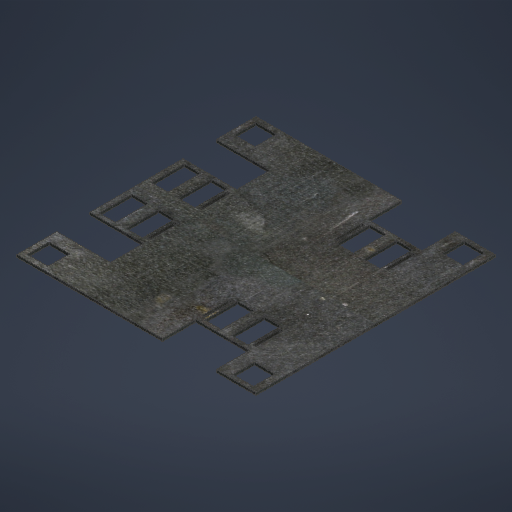
# Autodesk Inventor part: base2
Saved by Autodesk Inventor 2026.2 (Build 302298010, 298A)
## iProperties
Created: 2026-09-07
Part Number: base2
Material: Steel
Document SubType Name: Modeling
Designer: karol
Density: 7.85 g/cm^3
Appearance: Plate
Author: karol
Autodesk Inventor part; units mm, degrees
ref_plane "YZ Plane" through (0, 0, 0) normal (1, 0, 0) x (0, 1, 0)
ref_plane "XZ Plane" through (0, 0, 0) normal (0, 1, 0) x (-1, 0, 0)
ref_plane "XY Plane" through (0, 0, 0) normal (0, 0, 1) x (1, 0, 0)
sketch "Sketch1" plane through (0, 0, 0) normal (0, 1, 0) x (-1, 0, 0)
  line L0 (180, 90) -> (0, 90)
  line L1 (0, 90) -> (0, -90)
  line L2 (0, -90) -> (180, -90)
  line L3 (180, -90) -> (180, 90)
  line L4 (0, -0.2542) -> (0, 0)
  line L5 (0, 0) -> (0, 6.4289)
  line L6 (0, 0) -> (28.373, 0)
  line L7 (177, 0) -> (135, 0)
  line L8 (135, 0) -> (135, -7.5)
  line L9 (135, -7.5) -> (177, -7.5)
  line L10 (177, -7.5) -> (177, 0)
  line L11 (177, 0) -> (180, 0)
  line L12 (180, 0) -> (180, -35)
  line L13 (180, -35) -> (177, -35)
  line L14 (177, -35) -> (177, 0)
  line L15 (180, -35) -> (136.6, -35)
  line L16 (136.6, -35) -> (136.6, -32)
  line L17 (136.6, -32) -> (180, -32)
  line L18 (180, -32) -> (180, -35)
  line L19 (177, -7.5) -> (176, -7.5)
  line L20 (176, -7.5) -> (176, -32)
  line L21 (176, -32) -> (177, -32)
  line L22 (177, -32) -> (177, -7.5)
  line L23 (176, -7.5) -> (163.8, -7.5)
  line L24 (163.8, -7.5) -> (163.8, -32)
  line L25 (163.8, -32) -> (176, -32)
  line L26 (176, -32) -> (176, -7.5)
  line L27 (163.8, -7.5) -> (159.8, -7.5)
  line L28 (159.8, -7.5) -> (159.8, -32)
  line L29 (159.8, -32) -> (163.8, -32)
  line L30 (163.8, -32) -> (163.8, -7.5)
  line L31 (159.8, -7.5) -> (155.8, -7.5)
  line L32 (155.8, -7.5) -> (155.8, -32)
  line L33 (155.8, -32) -> (159.8, -32)
  line L34 (159.8, -32) -> (159.8, -7.5)
  line L35 (155.8, -7.5) -> (143.6, -7.5)
  line L36 (143.6, -7.5) -> (143.6, -32)
  line L37 (143.6, -32) -> (155.8, -32)
  line L38 (155.8, -32) -> (155.8, -7.5)
  line L39 (143.6, -7.5) -> (139.6, -7.5)
  line L40 (139.6, -7.5) -> (139.6, -32)
  line L41 (139.6, -32) -> (143.6, -32)
  line L42 (143.6, -32) -> (143.6, -7.5)
  line L43 (136.6, -35) -> (139.6, -35)
  line L44 (139.6, -35) -> (139.6, -32)
  line L45 (139.6, -32) -> (136.6, -32)
  line L46 (136.6, -32) -> (136.6, -35)
  line L47 (139.6, -35) -> (136.6, -35)
  line L48 (136.6, -35) -> (136.6, -60)
  line L49 (136.6, -60) -> (139.6, -60)
  line L50 (139.6, -60) -> (139.6, -35)
  line L51 (136.6, -60) -> (180, -60)
  line L52 (180, -60) -> (180, -63)
  line L53 (180, -63) -> (136.6, -63)
  line L54 (136.6, -63) -> (136.6, -60)
  line L55 (180, -63) -> (176, -63)
  line L56 (176, -63) -> (176, -90)
  line L57 (176, -90) -> (180, -90)
  line L58 (180, -90) -> (180, -63)
  line L59 (163.8, -7.5) -> (169.9, -7.5)
  line L60 (169.9, -7.5) -> (169.9, -32)
  line L61 (169.9, -32) -> (163.8, -32)
  line L62 (163.8, -32) -> (163.8, -7.5)
  line L63 (143.6, -7.5) -> (149.7, -7.5)
  line L64 (149.7, -7.5) -> (149.7, -32)
  line L65 (149.7, -32) -> (143.6, -32)
  line L66 (143.6, -32) -> (143.6, -7.5)
  line L67 (176, -90) -> (73.4, -90)
  line L68 (73.4, -90) -> (73.4, -86)
  line L69 (73.4, -86) -> (176, -86)
  line L70 (176, -86) -> (176, -90)
  line L71 (176, -86) -> (160.6, -86)
  line L72 (160.6, -86) -> (160.6, -69.8)
  line L73 (160.6, -69.8) -> (176, -69.8)
  line L74 (176, -69.8) -> (176, -86)
  line L75 (70.4, -90) -> (30, -90)
  line L76 (27, -90) -> (0, -90)
  line L77 (0, -90) -> (0, -87)
  line L78 (70.4, -90) -> (73.4, -90)
  line L79 (0, -90) -> (30, -90)
  line L80 (30, -90) -> (30, -87)
  line L81 (30, -87) -> (0, -87)
  line L82 (0, -87) -> (0, -90)
  line L83 (30, -87) -> (27, -87)
  line L84 (27, -87) -> (27, -65)
  line L85 (27, -65) -> (30, -65)
  line L86 (30, -65) -> (30, -87)
  line L87 (27, -65) -> (73.4, -65)
  line L88 (73.4, -65) -> (73.4, -62)
  line L89 (73.4, -62) -> (27, -62)
  line L90 (27, -62) -> (27, -65)
  line L91 (73.4, -62) -> (70.4, -62)
  line L92 (70.4, -62) -> (70.4, -90)
  line L93 (70.4, -90) -> (73.4, -90)
  line L94 (73.4, -90) -> (73.4, -62)
  line L95 (30, -90) -> (24, -90)
  line L96 (24, -90) -> (24, -84)
  line L97 (24, -84) -> (30, -84)
  line L98 (30, -84) -> (30, -90)
  line L99 (73.4, -62) -> (66.4, -62)
  line L100 (66.4, -62) -> (66.4, -37.5)
  line L101 (66.4, -37.5) -> (73.4, -37.5)
  line L102 (73.4, -37.5) -> (73.4, -62)
  line L103 (66.4, -37.5) -> (54.2, -37.5)
  line L104 (54.2, -37.5) -> (54.2, -62)
  line L105 (54.2, -62) -> (66.4, -62)
  line L106 (66.4, -62) -> (66.4, -37.5)
  line L107 (54.2, -37.5) -> (50.2, -37.5)
  line L108 (50.2, -37.5) -> (50.2, -62)
  line L109 (50.2, -62) -> (54.2, -62)
  line L110 (54.2, -62) -> (54.2, -37.5)
  line L111 (50.2, -37.5) -> (46.2, -37.5)
  line L112 (46.2, -37.5) -> (46.2, -62)
  line L113 (46.2, -62) -> (50.2, -62)
  line L114 (50.2, -62) -> (50.2, -37.5)
  line L115 (46.2, -37.5) -> (34, -37.5)
  line L116 (34, -37.5) -> (34, -62)
  line L117 (34, -62) -> (46.2, -62)
  line L118 (46.2, -62) -> (46.2, -37.5)
  line L119 (34, -37.5) -> (27, -37.5)
  line L120 (27, -37.5) -> (27, -62)
  line L121 (27, -62) -> (34, -62)
  line L122 (34, -62) -> (34, -37.5)
  line L123 (5, -87) -> (20.4, -87)
  line L124 (20.4, -87) -> (20.4, -70.8)
  line L125 (20.4, -70.8) -> (5, -70.8)
  line L126 (5, -70.8) -> (5, -87)
  line L127 (0, 90) -> (180, 90)
  line L128 (135, 7.5) -> (177, 7.5)
  line L129 (180, 35) -> (177, 35)
  line L130 (180, 35) -> (136.6, 35)
  line L131 (136.6, 35) -> (136.6, 32)
  line L132 (136.6, 32) -> (180, 32)
  line L133 (180, 32) -> (180, 35)
  line L134 (177, 7.5) -> (176, 7.5)
  line L135 (176, 7.5) -> (176, 32)
  line L136 (176, 32) -> (177, 32)
  line L137 (177, 32) -> (177, 7.5)
  line L138 (176, 7.5) -> (163.8, 7.5)
  line L139 (163.8, 7.5) -> (163.8, 32)
  line L140 (163.8, 32) -> (176, 32)
  line L141 (176, 32) -> (176, 7.5)
  line L142 (163.8, 7.5) -> (159.8, 7.5)
  line L143 (159.8, 7.5) -> (159.8, 32)
  line L144 (159.8, 32) -> (163.8, 32)
  line L145 (163.8, 32) -> (163.8, 7.5)
  line L146 (159.8, 7.5) -> (155.8, 7.5)
  line L147 (155.8, 7.5) -> (155.8, 32)
  line L148 (155.8, 32) -> (159.8, 32)
  line L149 (159.8, 32) -> (159.8, 7.5)
  line L150 (155.8, 7.5) -> (143.6, 7.5)
  line L151 (143.6, 7.5) -> (143.6, 32)
  line L152 (143.6, 32) -> (155.8, 32)
  line L153 (155.8, 32) -> (155.8, 7.5)
  line L154 (143.6, 7.5) -> (139.6, 7.5)
  line L155 (139.6, 7.5) -> (139.6, 32)
  line L156 (139.6, 32) -> (143.6, 32)
  line L157 (143.6, 32) -> (143.6, 7.5)
  line L158 (136.6, 35) -> (139.6, 35)
  line L159 (139.6, 35) -> (139.6, 32)
  line L160 (139.6, 32) -> (136.6, 32)
  line L161 (136.6, 32) -> (136.6, 35)
  line L162 (139.6, 35) -> (136.6, 35)
  line L163 (136.6, 35) -> (136.6, 60)
  line L164 (136.6, 60) -> (139.6, 60)
  line L165 (139.6, 60) -> (139.6, 35)
  line L166 (136.6, 60) -> (180, 60)
  line L167 (180, 60) -> (180, 63)
  line L168 (180, 63) -> (136.6, 63)
  line L169 (136.6, 63) -> (136.6, 60)
  line L170 (180, 63) -> (176, 63)
  line L171 (176, 63) -> (176, 90)
  line L172 (176, 90) -> (180, 90)
  line L173 (180, 90) -> (180, 63)
  line L174 (163.8, 7.5) -> (169.9, 7.5)
  line L175 (169.9, 7.5) -> (169.9, 32)
  line L176 (169.9, 32) -> (163.8, 32)
  line L177 (163.8, 32) -> (163.8, 7.5)
  line L178 (143.6, 7.5) -> (149.7, 7.5)
  line L179 (149.7, 7.5) -> (149.7, 32)
  line L180 (149.7, 32) -> (143.6, 32)
  line L181 (143.6, 32) -> (143.6, 7.5)
  line L182 (176, 90) -> (73.4, 90)
  line L183 (73.4, 90) -> (73.4, 86)
  line L184 (73.4, 86) -> (176, 86)
  line L185 (176, 86) -> (176, 90)
  line L186 (176, 86) -> (160.6, 86)
  line L187 (160.6, 86) -> (160.6, 69.8)
  line L188 (160.6, 69.8) -> (176, 69.8)
  line L189 (176, 69.8) -> (176, 86)
  line L190 (70.4, 90) -> (30, 90)
  line L191 (27, 90) -> (0, 90)
  line L192 (0, 90) -> (0, 87)
  line L193 (70.4, 90) -> (73.4, 90)
  line L194 (0, 90) -> (30, 90)
  line L195 (30, 90) -> (30, 87)
  line L196 (30, 87) -> (0, 87)
  line L197 (0, 87) -> (0, 90)
  line L198 (30, 87) -> (27, 87)
  line L199 (27, 87) -> (27, 65)
  line L200 (27, 65) -> (30, 65)
  line L201 (30, 65) -> (30, 87)
  line L202 (27, 65) -> (73.4, 65)
  line L203 (73.4, 65) -> (73.4, 62)
  line L204 (73.4, 62) -> (27, 62)
  line L205 (27, 62) -> (27, 65)
  line L206 (73.4, 62) -> (70.4, 62)
  line L207 (70.4, 62) -> (70.4, 90)
  line L208 (70.4, 90) -> (73.4, 90)
  line L209 (73.4, 90) -> (73.4, 62)
  line L210 (30, 90) -> (24, 90)
  line L211 (24, 90) -> (24, 84)
  line L212 (24, 84) -> (30, 84)
  line L213 (30, 84) -> (30, 90)
  line L214 (73.4, 62) -> (66.4, 62)
  line L215 (66.4, 62) -> (66.4, 37.5)
  line L216 (66.4, 37.5) -> (73.4, 37.5)
  line L217 (73.4, 37.5) -> (73.4, 62)
  line L218 (66.4, 37.5) -> (54.2, 37.5)
  line L219 (54.2, 37.5) -> (54.2, 62)
  line L220 (54.2, 62) -> (66.4, 62)
  line L221 (66.4, 62) -> (66.4, 37.5)
  line L222 (54.2, 37.5) -> (50.2, 37.5)
  line L223 (50.2, 37.5) -> (50.2, 62)
  line L224 (50.2, 62) -> (54.2, 62)
  line L225 (54.2, 62) -> (54.2, 37.5)
  line L226 (50.2, 37.5) -> (46.2, 37.5)
  line L227 (46.2, 37.5) -> (46.2, 62)
  line L228 (46.2, 62) -> (50.2, 62)
  line L229 (50.2, 62) -> (50.2, 37.5)
  line L230 (46.2, 37.5) -> (34, 37.5)
  line L231 (34, 37.5) -> (34, 62)
  line L232 (34, 62) -> (46.2, 62)
  line L233 (46.2, 62) -> (46.2, 37.5)
  line L234 (34, 37.5) -> (27, 37.5)
  line L235 (27, 37.5) -> (27, 62)
  line L236 (27, 62) -> (34, 62)
  line L237 (34, 62) -> (34, 37.5)
  line L238 (5, 87) -> (20.4, 87)
  line L239 (20.4, 87) -> (20.4, 70.8)
  line L240 (20.4, 70.8) -> (5, 70.8)
  line L241 (5, 70.8) -> (5, 87)
  line L242 (177, 7.5) -> (135, 7.5)
  line L243 (135, 7.5) -> (135, 0)
  line L244 (135, 0) -> (177, 0)
  line L245 (177, 0) -> (177, 7.5)
  point P0 (177, -3.75)
  point P1 (177, 3.75)
  point P2 (70.4, 65)
  point P3 (70.4, -65)
  dimension "d2" = 180
  dimension "d3" = 180
  dimension "d4" = 90
  dimension "d5" = 42
  dimension "d6" = 7.5
  dimension "d7" = 3
  dimension "d8" = 35
  dimension "d9" = 3
  dimension "d10" = 1
  dimension "d11" = 12.2
  dimension "d12" = 4
  dimension "d13" = 4
  dimension "d14" = 12.2
  dimension "d15" = 4
  dimension "d16" = 25
  dimension "d17" = 3
  dimension "d18" = 3
  dimension "d19" = 4
  dimension "d20" = 102.6
  dimension "d22" = 15.4
  dimension "d23" = 16.2
  dimension "d42" = 30
  dimension "d43" = 3
  dimension "d44" = 22
  dimension "d46" = 3
  dimension "d47" = 3
  dimension "d48" = 6
  dimension "d49" = 6
  dimension "d50" = 7
  dimension "d51" = 24.5
  dimension "d52" = 12.2
  dimension "d53" = 4
  dimension "d54" = 4
  dimension "d55" = 12.2
  dimension "d56" = 7
  dimension "d57" = 3
  dimension "d58" = 4
  dimension "d59" = 15.4
  dimension "d60" = 16.2
  dimension "d61" = 5
  constraints: 492 end point, 93 symmetric about line, 62 parallel, 35 point on line, 34 horizontal, 32 perpendicular, 5 midpoint, 1 collinear, 1 vertical
  measures "d2" distance of L2.end L1.end
  measures "d3" distance of L1.end L0.end
  measures "d4" distance between parallel lines of L0 L6
  measures "d5" distance of L9.end L8.end
  measures "d6" distance of L8.end L7.end
  measures "d7" distance from line of L3 point (177, -3.75)
  measures "d8" distance of L11.end L12.end
  measures "d9" distance of L15.end L16.end
  measures "d10" distance of L21.end L20.end
  measures "d11" distance of L25.end L24.end
  measures "d12" distance of L29.end L28.end
  measures "d13" distance of L33.end L32.end
  measures "d14" distance of L37.end L36.end
  measures "d15" distance of L41.end L40.end
  measures "d16" distance of L48.end L47.end
  measures "d17" distance of L51.end L52.end
  measures "d18" distance between parallel lines of L48 L50
  measures "d19" distance between parallel lines of L3 L56
  measures "d20" distance of L68.end L69.end
  measures "d22" distance of L72.end L73.end
  measures "d23" distance of L71.end L72.end
  measures "d42" distance of L81.end L80.end
  measures "d43" distance of L80.end L79.end
  measures "d44" distance of L83.end L84.end
  measures "d46" distance of L88.end L87.end
  measures "d47" distance of L93.end L92.end
  measures "d48" distance of L96.end L97.end
  measures "d49" distance of L95.end L96.end
  measures "d50" distance of L100.end L101.end
  measures "d51" distance of L99.end L100.end
  measures "d52" distance of L105.end L104.end
  measures "d53" distance of L109.end L108.end
  measures "d54" distance of L113.end L112.end
  measures "d55" distance of L117.end L116.end
  measures "d56" distance between parallel lines of L116 L120
  measures "d57" distance between parallel lines of L98 L84
  measures "d58" distance between parallel lines of L67 L69
  measures "d59" distance of L125.end L124.end
  measures "d60" distance of L124.end L123.end
  measures "d61" distance between parallel lines of L126 L1
extrude "Extrusion1" add sketch "Sketch1" along normal blind 2 contours L3 L168 L171 L0 | L171 L184 L183 L0 | L3 L166 L164 L169 L168 | L183 L209 L202 L207 L0 | L168 L169 L163 L131 L132 L155 L128 L243 L8 L9 L40 L17 L16 L48 L54 L53 L56 L73 L72 L69 L94 L88 L102 L101 L103 L107 L111 L115 L119 L120 L90 L84 L97 L96 L81 L124 L125 L126 L1 L196 L241 L240 L239 L211 L212 L199 L205 L235 L234 L230 L226 L222 L218 L216 L217 L203 L209 L184 L187 L188 L171 | L3 L132 L159 L130 L129 | L165 L130 L163 L164 | L195 L196 L211 L0 | L207 L204 L205 L200 L202 | L202 L203 L204 L207 | L3 L11 L245 L137 L132 | L159 L132 L131 L130 | L201 L212 L199 L196 | L200 L199 L212 L201 | L204 L217 L216 L215 | L3 L17 L14 L10 L11 | L137 L128 L135 L132 | L132 L151 L128 L155 | L211 L196 L1 L0 | L199 L212 L211 L196 | L3 L13 L14 L17 | L10 L9 L8 L7 | L7 L243 L128 L245 | L204 L231 L234 L235 | L219 L222 L223 L204 | L17 L20 L9 L14 | L14 L15 L44 L17 | L223 L226 L227 L204 | L3 L53 L54 L49 L51 | L139 L128 L143 L132 | L132 L143 L128 L147 | L3 L2 L56 L53 | L49 L48 L15 L50 | L15 L16 L17 L44 | L9 L36 L17 L40 | L17 L28 L9 L24 | L2 L68 L69 L56 | L17 L32 L9 L28 | L81 L96 L2 L1 | L2 L92 L87 L94 L68 | L96 L81 L80 L2 | L92 L89 L88 L87 | L87 L85 L90 L89 L92 | L96 L97 L84 L81 | L81 L84 L97 L86 | L86 L97 L84 L85 | L89 L100 L101 L102 | L120 L119 L116 L89 | L89 L108 L107 L104 | L89 L112 L111 L108
sketch "Sketch2" plane through (0, 0, 0) normal (0, -1, 0) x (1, 0, 0)
  line L0 (-143.6, -7.5) -> (-155.8, -7.5) projected
  line L1 (-143.6, -7.5) -> (-141.6, -7.5)
  line L2 (-141.6, -7.5) -> (-141.6, -32)
  line L3 (-141.6, -32) -> (-143.6, -32)
  line L4 (-143.6, -32) -> (-143.6, -7.5)
  line L5 (-143.6, 7.5) -> (-143.6, 32) projected
  line L6 (-143.6, 32) -> (-141.6, 32)
  line L7 (-141.6, 32) -> (-141.6, 7.5)
  line L8 (-141.6, 7.5) -> (-143.6, 7.5)
  line L9 (-143.6, 7.5) -> (-143.6, 32)
  line L10 (-141.6, 32) -> (-139.6, 32)
  line L11 (-139.6, 32) -> (-139.6, 7.5)
  line L12 (-139.6, 7.5) -> (-141.6, 7.5)
  line L13 (-141.6, 7.5) -> (-141.6, 32)
  line L14 (-141.6, -7.5) -> (-139.6, -7.5)
  line L15 (-139.6, -7.5) -> (-139.6, -32)
  line L16 (-139.6, -32) -> (-141.6, -32)
  line L17 (-141.6, -32) -> (-141.6, -7.5)
  line L18 (-66.4, 62) -> (-66.4, 37.5) projected
  line L19 (-66.4, 62) -> (-68.4, 62)
  line L20 (-68.4, 62) -> (-68.4, 37.5)
  line L21 (-68.4, 37.5) -> (-66.4, 37.5)
  line L22 (-66.4, 37.5) -> (-66.4, 62)
  line L23 (-34, 37.5) -> (-34, 62) projected
  line L24 (-34, 62) -> (-32, 62)
  line L25 (-32, 62) -> (-32, 37.5)
  line L26 (-32, 37.5) -> (-34, 37.5)
  line L27 (-34, 37.5) -> (-34, 62)
  line L28 (-32, 62) -> (-30, 62)
  line L29 (-30, 62) -> (-30, 37.5)
  line L30 (-30, 37.5) -> (-32, 37.5)
  line L31 (-32, 37.5) -> (-32, 62)
  line L32 (-68.4, 62) -> (-70.4, 62)
  line L33 (-70.4, 62) -> (-70.4, 37.5)
  line L34 (-70.4, 37.5) -> (-68.4, 37.5)
  line L35 (-68.4, 37.5) -> (-68.4, 62)
  line L36 (-34, -37.5) -> (-46.2, -37.5) projected
  line L37 (-34, -37.5) -> (-32, -37.5)
  line L38 (-32, -37.5) -> (-32, -62)
  line L39 (-32, -62) -> (-34, -62)
  line L40 (-34, -62) -> (-34, -37.5)
  line L41 (-32, -62) -> (-30, -62)
  line L42 (-30, -62) -> (-30, -37.5)
  line L43 (-30, -37.5) -> (-32, -37.5)
  line L44 (-32, -37.5) -> (-32, -62)
  line L45 (-54.2, -37.5) -> (-66.4, -37.5) projected
  line L46 (-66.4, -37.5) -> (-68.4, -37.5)
  line L47 (-68.4, -37.5) -> (-68.4, -62)
  line L48 (-68.4, -62) -> (-66.4, -62)
  line L49 (-66.4, -62) -> (-66.4, -37.5)
  line L50 (-68.4, -62) -> (-70.4, -62)
  line L51 (-70.4, -62) -> (-70.4, -37.5)
  line L52 (-70.4, -37.5) -> (-68.4, -37.5)
  line L53 (-68.4, -37.5) -> (-68.4, -62)
  line L54 (-70.4, -37.5) -> (-66.4, -37.5)
  line L55 (-66.4, -37.5) -> (-66.4, -39.5)
  line L56 (-66.4, -39.5) -> (-70.4, -39.5)
  line L57 (-70.4, -39.5) -> (-70.4, -37.5)
  line L58 (-66.4, -62) -> (-70.4, -62)
  line L59 (-70.4, -62) -> (-70.4, -60)
  line L60 (-70.4, -60) -> (-66.4, -60)
  line L61 (-66.4, -60) -> (-66.4, -62)
  line L62 (-34, -62) -> (-30, -62)
  line L63 (-30, -62) -> (-30, -60)
  line L64 (-30, -60) -> (-34, -60)
  line L65 (-34, -60) -> (-34, -62)
  line L66 (-34, -37.5) -> (-30, -37.5)
  line L67 (-30, -37.5) -> (-30, -39.5)
  line L68 (-30, -39.5) -> (-34, -39.5)
  line L69 (-34, -39.5) -> (-34, -37.5)
  line L70 (-143.6, -32) -> (-139.6, -32)
  line L71 (-139.6, -32) -> (-139.6, -30)
  line L72 (-139.6, -30) -> (-143.6, -30)
  line L73 (-143.6, -30) -> (-143.6, -32)
  line L74 (-143.6, -7.5) -> (-139.6, -7.5)
  line L75 (-139.6, -7.5) -> (-139.6, -9.5)
  line L76 (-139.6, -9.5) -> (-143.6, -9.5)
  line L77 (-143.6, -9.5) -> (-143.6, -7.5)
  line L78 (-143.6, 32) -> (-139.6, 32)
  line L79 (-139.6, 32) -> (-139.6, 30)
  line L80 (-139.6, 30) -> (-143.6, 30)
  line L81 (-143.6, 30) -> (-143.6, 32)
  line L82 (-139.6, 7.5) -> (-143.6, 7.5)
  line L83 (-143.6, 7.5) -> (-143.6, 9.5)
  line L84 (-143.6, 9.5) -> (-139.6, 9.5)
  line L85 (-139.6, 9.5) -> (-139.6, 7.5)
  line L86 (-70.4, 62) -> (-66.4, 62)
  line L87 (-66.4, 62) -> (-66.4, 60)
  line L88 (-66.4, 60) -> (-70.4, 60)
  line L89 (-70.4, 60) -> (-70.4, 62)
  line L90 (-66.4, 37.5) -> (-70.4, 37.5)
  line L91 (-70.4, 37.5) -> (-70.4, 39.5)
  line L92 (-70.4, 39.5) -> (-66.4, 39.5)
  line L93 (-66.4, 39.5) -> (-66.4, 37.5)
  line L94 (-34, 37.5) -> (-30, 37.5)
  line L95 (-30, 37.5) -> (-30, 39.5)
  line L96 (-30, 39.5) -> (-34, 39.5)
  line L97 (-34, 39.5) -> (-34, 37.5)
  line L98 (-34, 62) -> (-30, 62)
  line L99 (-30, 62) -> (-30, 60)
  line L100 (-30, 60) -> (-34, 60)
  line L101 (-34, 60) -> (-34, 62)
  point P0 (0, 0)
  point P1 (-31, -62)
  point P2 (-141.6, 9.5)
  point P3 (-141.6, 30)
  point P4 (-141.6, -9.5)
  point P5 (-141.6, -30)
  point P6 (-68.4, -60)
  point P7 (-68.4, -39.5)
  point P8 (-32, -39.5)
  point P9 (-32, -60)
  point P10 (-32, 60)
  point P11 (-32, 39.5)
  point P12 (-68.4, 39.5)
  point P13 (-68.4, 60)
  dimension "d64" = 2
  dimension "d65" = 2
  dimension "d66" = 2
  dimension "d67" = 2
  dimension "d68" = 2
  dimension "d69" = 2
  dimension "d70" = 2
  dimension "d71" = 2
  dimension "d72" = 2
  dimension "d73" = 2
  dimension "d74" = 2
  dimension "d75" = 2
  dimension "d76" = 2
  dimension "d77" = 2
  dimension "d78" = 2
  dimension "d79" = 2
  dimension "d80" = 2
  dimension "d81" = 2
  dimension "d82" = 2
  dimension "d83" = 2
  dimension "d84" = 2
  dimension "d85" = 2
  dimension "d86" = 2
  constraints: 192 end point, 48 parallel, 24 horizontal, 24 perpendicular, 21 point on line, 1 midpoint
  measures "d64" distance of L2.end L3.end
  measures "d65" distance of L7.end L8.end
  measures "d66" distance of L11.end L12.end
  measures "d67" distance of L15.end L16.end
  measures "d68" distance of L21.end L20.end
  measures "d69" distance of L25.end L26.end
  measures "d70" distance of L29.end L30.end
  measures "d71" distance of L34.end L33.end
  measures "d72" distance of L38.end L39.end
  measures "d73" distance of L43.end L42.end
  measures "d74" distance of L48.end L47.end
  measures "d75" distance of L51.end L52.end
  measures "d76" distance of L54.end L55.end
  measures "d77" distance of L58.end L59.end
  measures "d78" distance from line of point (-31, -62) L64
  measures "d79" distance of L71.end L70.end
  measures "d80" distance of L74.end L75.end
  measures "d81" distance of L78.end L79.end
  measures "d82" distance of L82.end L83.end
  measures "d83" distance of L86.end L87.end
  measures "d84" distance of L90.end L91.end
  measures "d85" distance of L95.end L94.end
  measures "d86" distance of L98.end L99.end
extrude "Extrusion2" cut sketch "Sketch2" against normal blind 2 contours L76 L15 L72 L2 | L7 L80 L11 L84 | L20 L92 L33 L88 | L25 L100 L29 L96 | L68 L42 L64 L38 | L47 L60 L51 L56
body "Solid1"
